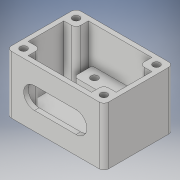
# Autodesk Inventor part: Caixa
Saved by Autodesk Inventor 2019 (Build 230136000, 136)
## iProperties
Created: 2021-05-27
Part Number: Caixa
Material: Generic
Document SubType Name: Modeling
Designer: hoope
Density: 1 g/cm^3
Appearance: Default
Author: hoope
Autodesk Inventor part; units mm, degrees
ref_plane "YZ Plane" through (0, 0, 0) normal (1, 0, 0) x (0, 1, 0)
ref_plane "XZ Plane" through (0, 0, 0) normal (0, 1, 0) x (-1, 0, 0)
ref_plane "XY Plane" through (0, 0, 0) normal (0, 0, 1) x (1, 0, 0)
sketch "Esboço1" plane through (0, 0, 0) normal (0, 1, 0) x (-1, 0, 0)
  line L0 (0, 0) -> (42, 0)
  line L1 (42, 0) -> (42, 30)
  line L2 (42, 30) -> (0, 30)
  line L3 (0, 30) -> (0, 0)
  dimension "d0" = 42
  dimension "d1" = 30
  constraints: 8 end point, 2 parallel, 1 horizontal, 1 perpendicular
  measures "d0" distance of L2.end L1.end
  measures "d1" distance of L1.end L0.end
extrude "Extrusão1" add sketch "Esboço1" along normal blind 25
shell "Casca1" thickness 2 removed faces 1 at (-14, 25, 20)
sketch "Esboço2" plane through (-42, 0, 30) normal (0, 0, 1) x (1, 0, 0)
  arc A0 (12, 17.15) -> (12, 7.85) centre (12, 12.5) ccw
  line L0 (0, 25) -> (42, 25) projected
  arc A1 (30, 7.85) -> (30, 17.15) centre (30, 12.5) ccw
  line L1 (42, 0) -> (42, 25) projected
  line L2 (12, 17.15) -> (30, 17.15)
  line L3 (30, 7.85) -> (12, 7.85)
  dimension "d5" = 9.3
  dimension "d6" = 12.5
  dimension "d7" = 9.3
  dimension "d8" = 18
  dimension "d9" = 12
  constraints: 4 end point, 4 point on circle, 2 centre point, 1 horizontal, 1 parallel
  measures "d5" diameter of A0
  measures "d6" distance from line of L0 A0.centre
  measures "d7" diameter of A1
  measures "d8" distance of A1.centre A0.centre
  measures "d9" distance from line of L1 A1.centre
extrude "Extrusão2" cut sketch "Esboço2" against normal blind 10
sketch "Esboço3" plane through (-40, 2, 2) normal (0, 1, 0) x (1, 0, 0)
  line L0 (38, 0) -> (0, 0) projected
  line L1 (0, 0) -> (5.3, 0)
  line L2 (5.3, 0) -> (5.3, -5.3)
  line L3 (5.3, -5.3) -> (0, -5.3)
  line L4 (0, -5.3) -> (0, 0)
  line L5 (38, 0) -> (32.7, 0)
  line L6 (32.7, 0) -> (32.7, -5.3)
  line L7 (32.7, -5.3) -> (38, -5.3)
  line L8 (38, -5.3) -> (38, 0)
  line L9 (38, -26) -> (32.7, -26)
  line L10 (32.7, -26) -> (32.7, -20.7)
  line L11 (32.7, -20.7) -> (38, -20.7)
  line L12 (38, -20.7) -> (38, -26)
  line L13 (38, -26) -> (0, -26) projected
  line L14 (0, -26) -> (5.3, -26)
  line L15 (5.3, -26) -> (5.3, -20.7)
  line L16 (5.3, -20.7) -> (0, -20.7)
  line L17 (0, -20.7) -> (0, -26)
  point P0 (40, 2)
  dimension "d12" = 5.3
  dimension "d13" = 5.3
  dimension "d14" = 5.3
  dimension "d15" = 5.3
  dimension "d16" = 5.3
  dimension "d17" = 5.3
  dimension "d18" = 5.3
  dimension "d19" = 5.3
  constraints: 32 end point, 8 parallel, 4 horizontal, 4 perpendicular
  measures "d12" distance of L2.end L3.end
  measures "d13" distance of L1.end L2.end
  measures "d14" distance of L7.end L6.end
  measures "d15" distance of L6.end L5.end
  measures "d16" distance of L10.end L11.end
  measures "d17" distance of L9.end L10.end
  measures "d18" distance of L16.end L15.end
  measures "d19" distance of L15.end L14.end
extrude "Extrusão3" add sketch "Esboço3" along normal blind 23
sketch "Esboço4" plane through (-34.7, 2, 2) normal (0, 1, 0) x (1, 0, 0)
  circle A0 centre (6.62, -4) radius 1.555
  circle A1 centre (22.18, -4) radius 1.555
  line L0 (27.4, 0) -> (27.4, -5.3) projected
  line L1 (0, -5.3) -> (0, 0) projected
  line L2 (0, 0) -> (27.4, 0) projected
  line L3 (27.4, 0) -> (0, 0) projected
  line L4 (1.7, 0) -> (25.7, 0)
  line L5 (25.7, 0) -> (25.7, -8)
  line L6 (25.7, -8) -> (1.7, -8)
  line L7 (1.7, -8) -> (1.7, 0)
  point P0 (34.7, 2)
  dimension "d22" = 3.11
  dimension "d23" = 3.11
  dimension "d24" = 15.56
  dimension "d25" = 5.22
  dimension "d27" = 4
  dimension "d28" = 4
  dimension "d33" = 24
  dimension "d34" = 8
  dimension "d35" = 1.7
  constraints: 8 end point, 2 centre point, 2 parallel, 1 horizontal, 1 perpendicular, 1 point on line
  measures "d22" diameter of A0
  measures "d23" diameter of A1
  measures "d24" distance of A1.centre A0.centre
  measures "d25" distance from line of L0 A1.centre
  measures "d27" distance from line of L2 A0.centre
  measures "d28" distance from line of L2 A1.centre
  measures "d33" distance between parallel lines of L5 L7
  measures "d34" distance between parallel lines of L4 L6
  measures "d35" distance between parallel lines of L0 L5
extrude "Extrusão4" add sketch "Esboço4" along normal blind 3
sketch "Esboço5" plane through (-34.7, 5, 2) normal (0, 1, 0) x (1, 0, 0)
  circle A0 centre (6.62, -4) radius 1.555 projected
  circle A1 centre (6.62, -4) radius 1.5
  circle A2 centre (22.18, -4) radius 1.555 projected
  circle A3 centre (22.18, -4) radius 1.5
  line L0 (27.4, 0) -> (25.7, 0) projected
  line L1 (1.7, -8) -> (25.7, -8)
  line L2 (25.7, -8) -> (25.7, 0)
  line L3 (25.7, 0) -> (1.7, 0)
  line L4 (1.7, 0) -> (1.7, -8)
  point P0 (34.7, 2)
  dimension "d38" = 3
  dimension "d39" = 3
  constraints: 8 end point, 2 centre point, 2 coincident, 2 parallel, 1 horizontal, 1 perpendicular
  measures "d38" diameter of A1
  measures "d39" diameter of A3
extrude "Extrusão5" add sketch "Esboço5" along normal blind 4 contours L4 L3 L2 L1
chamfer "Chanfro1" distance 1 angle 45 2 edges at (-33, 5.5, 10) (-9, 5.5, 10)
sketch "Esboço6" plane through (0, 25, 0) normal (0, 1, 0) x (1, 0, 0)
  circle A0 centre (-38.35, -3.65) radius 1.505
  line L0 (0, 0) -> (-42, 0) projected
  line L1 (-42, 0) -> (-42, -30) projected
  circle A1 centre (-3.65, -26.35) radius 1.505
  line L2 (0, -30) -> (0, 0) projected
  line L3 (-42, -30) -> (0, -30) projected
  circle A2 centre (-3.65, -3.65) radius 1.505
  circle A3 centre (-38.35, -26.35) radius 1.505
  dimension "d48" = 3.01
  dimension "d49" = 3.65
  dimension "d50" = 3.65
  dimension "d51" = 3.01
  dimension "d52" = 3.65
  dimension "d53" = 3.65
  dimension "d54" = 3.01
  dimension "d55" = 3.01
  dimension "d56" = 3.65
  dimension "d57" = 3.65
  dimension "d65" = 3.65
  dimension "d66" = 3.65
  constraints: 4 centre point
  measures "d48" diameter of A0
  measures "d49" distance from line of L0 A0.centre
  measures "d50" distance from line of L1 A0.centre
  measures "d51" diameter of A1
  measures "d52" distance from line of L2 A1.centre
  measures "d53" distance from line of L3 A1.centre
  measures "d54" diameter of A2
  measures "d55" diameter of A3
  measures "d56" distance from line of L1 A3.centre
  measures "d57" distance from line of L3 A3.centre
  measures "d65" distance from line of L0 A2.centre
  measures "d66" distance from line of L2 A2.centre
extrude "Extrusão6" cut sketch "Esboço6" against normal blind 15 contours A0 | A1 | A2 | A3
fillet "Arredondamento1" radius 2 4 edges at (-42, 12.5, 30) (0, 12.5, 30) (0, 12.5, 0) (-42, 12.5, 0)
fillet "Arredondamento2" radius 2 4 edges at (-34.7, 13.5, 7.3) (-7.3, 13.5, 7.3) (-34.7, 13.5, 22.7) (-7.3, 13.5, 22.7)
